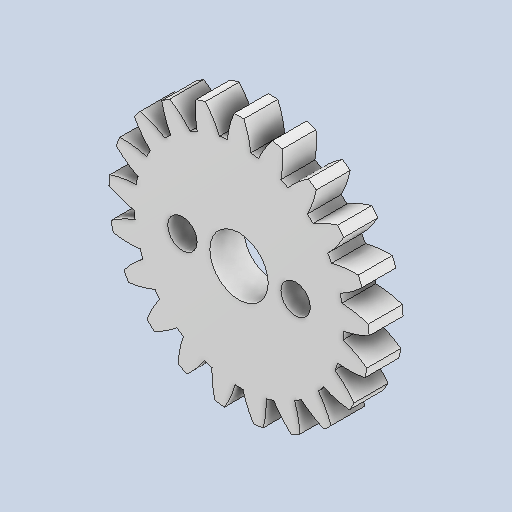
# Autodesk Inventor part: 平歯車1
Saved by Autodesk Inventor 2025.2 (Build 292293000, 293)
## iProperties
CustomPartVersion: 1
Created: 2025-01-07
Part Number: 平歯車1
Material: ABS プラスチック
Document SubType Name: Modeling
Designer: haruy
Categories: <?xml version="1.0" encoding="UTF-16"?> <MemberInstance><Categories><FamilyTemplate><FamilyTemplateParameter ValueType="xs:double" Id="1" ObjectReferenceKey="da_z" ObjectType="kUserParameterObject"/><FamilyTemplateParameter ValueType="xs:double" Id="2" ObjectReferenceKey="da_b" ObjectType="kUserParameterObject"/><FamilyTemplateParameter ValueType="xs:double" Id="3" ObjectReferenceKey="da_beta" ObjectType="kUserParameterObject"/><FamilyTemplateParameter ValueType="xs:double" Id="4" ObjectReferenceKey="da_da" ObjectType="kUserParameterObject"/><FamilyTemplateParameter ValueType="xs:double" Id="5" ObjectReferenceKey="da_aw" ObjectType="kUserParameterObject"/><FamilyTemplateParameter ValueType="xs:string" Id="6" ObjectReferenceKey="EAIAABAAAACIAQAAAAAAAIAAAAAAAAAA" ObjectType="83910656" SubObjectId="SurfaceGeometry"/></FamilyTemplate><ParamToTemplateMap><ParamToTemplate CategoryParameter="//CategoryParameter[@InternalName='046C89C9-8512-4d59-83FE-43B91F4F132A']" TemplateParameter="1"/><ParamToTemplate CategoryParameter="//CategoryParameter[@InternalName='2552DF32-E462-4b46-AEBF-C6C7768E72AC']" TemplateParameter="2"/><ParamToTemplate CategoryParameter="//CategoryParameter[@InternalName='C9EE641D-15FC-4fae-A226-E94C4372FDD7']" TemplateParameter="3"/><ParamToTemplate><ParamToTemplate CategoryParameter="//CategoryParameter[@InternalName='00B6519A-459B-49c7-AD84-2E56D39A5744']" ConstantValue="0.000000"/></ParamToTemplate><ParamToTemplate><ParamToTemplate CategoryParameter="//CategoryParameter[@InternalName='04B31F0E-C7A6-4894-AA32-9629BEFACF47']" ConstantValue="1.000000"/></ParamToTemplate><ParamToTemplate><ParamToTemplate CategoryParameter="//CategoryParameter[@InternalName='43CBEC2E-7847-49e7-A936-2F7889FCB2D9']" ConstantValue="0.250000"/></ParamToTemplate><ParamToTemplate><ParamToTemplate CategoryParameter="//CategoryParameter[@InternalName='B1EFC894-105D-4ebd-86BF-FA20ED196853']" ConstantValue="0.350000"/></ParamToTemplate><ParamToTemplate><ParamToTemplate CategoryParameter="//CategoryParameter[@InternalName='51175063-3D10-4879-93E8-6246FE8B403D']" ConstantValue="2060000000.000000"/></ParamToTemplate><ParamToTemplate><ParamToTemplate CategoryParameter="//CategoryParameter[@InternalName='A3A52E27-4454-46a9-B0BD-C932399B70AF']" ConstantValue="0.300000"/></ParamToTemplate><ParamToTemplate><ParamToTemplate CategoryParameter="//CategoryParameter[@InternalName='91B76062-C214-41d9-B1B9-14D2AB99603D']" ConstantValue="0.200000"/></ParamToTemplate><ParamToTemplate><ParamToTemplate CategoryParameter="//CategoryParameter[@InternalName='374E806E-8B8A-4dda-A9AA-1039D6500AD2']" ConstantValue="5.000000"/></ParamToTemplate><ParamToTemplate><ParamToTemplate CategoryParameter="//CategoryParameter[@InternalName='2D373A89-B862-43d6-8D0B-0CBF12AB9F6C']" ConstantValue="0.349066"/></ParamToTemplate><ParamToTemplate CategoryParameter="//CategoryParameter[@InternalName='37777632-D6A2-4fac-9D53-DB8ACD95C989']" TemplateParameter="4"/><ParamToTemplate CategoryParameter="//CategoryParameter[@InternalName='FD1017F1-B727-4f7e-9707-0F86F1FF9423']" TemplateParameter="5"/><ParamToTemplate><ParamToTemplate CategoryParameter="//CategoryParameter[@InternalName='9E1B4470-B2D3-4ff1-B813-535BB4CDF51A']" ConstantValue="3520000.000000"/></ParamToTemplate><ParamToTemplate><ParamToTemplate CategoryParameter="//CategoryParameter[@InternalName='F8452263-BFF6-458c-9FB1-07C4B99E95CD']" ConstantValue="11400000.000000"/></ParamToTemplate><ParamToTemplate><ParamToTemplate CategoryParameter="//CategoryParameter[@InternalName='3E3BB259-FD49-497f-8171-6EBC954A3479']" ConstantValue="2.000000"/></ParamToTemplate><ParamToTemplate CategoryParameter="//CategoryParameter[@InternalName='27C3BAF2-7550-4e4b-AE2C-0DB134B7D9B7']" TemplateParameter="6"/></ParamToTemplateMap><Category DisplayName="Gear" InternalName="DC85795E-93AB-48d5-8EEE-5A27447B64BD" Mnemonic="Gear"><CategoryParameter DisplayName="z" InternalName="046C89C9-8512-4d59-83FE-43B91F4F132A" Mnemonic="z"/><CategoryParameter DisplayName="b" InternalName="2552DF32-E462-4b46-AEBF-C6C7768E72AC" Mnemonic="b"/><CategoryParameter DisplayName="||b|" InternalName="C9EE641D-15FC-4fae-A226-E94C4372FDD7" Mnemonic="beta"/><CategoryParameter DisplayName="x" InternalName="00B6519A-459B-49c7-AD84-2E56D39A5744" Mnemonic="x"/><CategoryParameter DisplayName="a*" InternalName="04B31F0E-C7A6-4894-AA32-9629BEFACF47" Mnemonic="a"/><CategoryParameter DisplayName="c*" InternalName="43CBEC2E-7847-49e7-A936-2F7889FCB2D9" Mnemonic="c"/><CategoryParameter DisplayName="r|.f|*" InternalName="B1EFC894-105D-4ebd-86BF-FA20ED196853" Mnemonic="rf"/><CategoryParameter DisplayName="E" InternalName="51175063-3D10-4879-93E8-6246FE8B403D" Mnemonic="E"/><CategoryParameter DisplayName="||m|" InternalName="A3A52E27-4454-46a9-B0BD-C932399B70AF" Mnemonic="mi"/><Category DisplayName="SpurGear" InternalName="26C5A22E-A91E-4dfd-A3B3-23CCAFAE1764" Mnemonic="SpurGear"><CategoryParameter DisplayName="m" InternalName="91B76062-C214-41d9-B1B9-14D2AB99603D" Mnemonic="m"/><CategoryParameter DisplayName="P" InternalName="374E806E-8B8A-4dda-A9AA-1039D6500AD2" Mnemonic="PP"/><CategoryParameter DisplayName="||a|" InternalName="2D373A89-B862-43d6-8D0B-0CBF12AB9F6C" Mnemonic="alpha"/><CategoryParameter DisplayName="d|.a|" InternalName="37777632-D6A2-4fac-9D53-DB8ACD95C989" Mnemonic="da"/><CategoryParameter DisplayName="a|.w|" InternalName="FD1017F1-B727-4f7e-9707-0F86F1FF9423" Mnemonic="aw"/><CategoryParameter DisplayName="||s||.Flim|" InternalName="9E1B4470-B2D3-4ff1-B813-535BB4CDF51A" Mnemonic="sFlim"/><CategoryParameter DisplayName="||s||.Hlim|" InternalName="F8452263-BFF6-458c-9FB1-07C4B99E95CD" Mnemonic="sHlim"/><CategoryParameter DisplayName="タイプ" InternalName="3E3BB259-FD49-497f-8171-6EBC954A3479" Mnemonic="type"/><CategoryParameter DisplayName="PitchDiameter" InternalName="27C3BAF2-7550-4e4b-AE2C-0DB134B7D9B7" Mnemonic="IDS_PITCHDIAM"/></Category></Category></Categories></MemberInstance>
Density: 1.06 g/cm^3
Appearance: 滑らか - 白
Mass: 64.8659 g
Surface Area: 43.5022 cm^2
Volume: 8.26317 cm^3
Author: haruy
Autodesk Inventor part; units mm, degrees
sketch "Sketch1" plane through (0, 0, 0) normal (0, 0, 1) x (1, 0, 0)
  circle A0 centre (0, 0) radius 23
  dimension "d0" = 46
  constraints: 1 centre point
  measures "d0" diameter of A0
extrude "Extrusion1" add sketch "Sketch1" along normal blind 6
ref_plane "Work Plane2" through (0, 0, 3) normal (0, 0, 1) x (1, 0, 0)
sketch "Sketch2" plane through (0, 0, 0) normal (0, 0, -1) x (-1, 0, 0)
  circle A0 centre (0, 0) radius 23 projected
  circle A1 centre (0, 0) radius 21
  dimension "d3" = 42
  constraints: 1 centre point, 1 coincident
  measures "d3" diameter of A1
surface extrude "ピッチ円直径" sketch "Sketch2" against normal through all shown no curves A1
ref_plane "Work Plane8" through (0, 0, 0) normal (0.9888308, 0.1490423, 0) x (0, 0, 1)
ref_plane "Work Plane9" through (0, 0, 0) normal (1, 0, 0) x (0, 1, 0)
spur gear teeth "平歯車" teeth 21 pitch diameter 42 tip diameter 46 root diameter 37 face width 6 start plane through (0, 0, 0) normal (0, 0, -1) x (-1, 0, 0)
sketch "スケッチ3" plane through (0, 0, 6) normal (0, 0, 1) x (1, 0, 0)
  circle A0 centre (0, 0) radius 5.15
  circle A1 centre (0, 0) radius 10
  circle A2 centre (-10, 0) radius 2.6
  circle A3 centre (10, 0) radius 2.6
  dimension "d50" = 20
  dimension "d49" = 10.3
  dimension "d51" = 5.2
  dimension "d54" = 360
  constraints: 3 centre point, 2 coincident, 1 horizontal alignment, 7 other
  measures "d49" diameter of A0
  measures "d51" diameter of A2
extrude "押し出し2" cut sketch "スケッチ3" against normal blind 10 contours A0 | A1 A3 | A1 A3 | A2 A1 | A1 A2
sketch "スケッチ4" plane through (0, 0, 6) normal (0, 0, 1) x (1, 0, 0)
  circle A0 centre (10, 0) radius 2.6 projected
  circle A1 centre (-10, 0) radius 2.6 projected
  circle A2 centre (0, 0) radius 5.15 projected
  arc A3 (-5.9528, 22.2163) -> (-7.5964, 21.7093) centre (0, 0) ccw projected
  arc A4 (-7.5964, 21.7093) -> (-7.398, 16.9564) centre (9.3156, 20.0347) ccw projected
  arc A5 (-7.398, 16.9564) -> (-8.6445, 16.3561) centre (0, 0) ccw projected
  arc A6 (-8.6445, 16.3561) -> (-12.2367, 19.4747) centre (-21.472, 5.2082) ccw projected
  arc A7 (-12.2367, 19.4747) -> (-13.6579, 18.5057) centre (0, 0) ccw projected
  arc A8 (-13.6579, 18.5057) -> (-12.0673, 14.0225) centre (2.9964, 21.8905) ccw projected
  arc A9 (-12.0673, 14.0225) -> (-13.0815, 13.0815) centre (0, 0) ccw projected
  arc A10 (-13.0815, 13.0815) -> (-17.4333, 15.0026) centre (-22.0532, -1.3521) ccw projected
  arc A11 (-17.4333, 15.0026) -> (-18.5057, 13.6579) centre (0, 0) ccw projected
  arc A12 (-18.5057, 13.6579) -> (-15.6644, 9.8426) centre (-3.5891, 21.8011) ccw projected
  arc A13 (-15.6644, 9.8426) -> (-16.3561, 8.6445) centre (0, 0) ccw projected
  arc A14 (-16.3561, 8.6445) -> (-21.0809, 9.1975) centre (-20.6749, -7.7924) ccw projected
  arc A15 (-21.0809, 9.1975) -> (-21.7093, 7.5964) centre (0, 0) ccw projected
  arc A16 (-21.7093, 7.5964) -> (-17.8696, 4.7882) centre (-9.8556, 19.7747) ccw projected
  arc A17 (-17.8696, 4.7882) -> (-18.1775, 3.4394) centre (0, 0) ccw projected
  arc A18 (-18.1775, 3.4394) -> (-22.8554, 2.5752) centre (-17.4595, -13.5402) ccw projected
  arc A19 (-22.8554, 2.5752) -> (-22.9839, 0.86) centre (0, 0) ccw projected
  arc A20 (-22.9839, 0.86) -> (-18.4871, -0.6917) centre (-15.2464, 15.9912) ccw projected
  arc A21 (-18.4871, -0.6917) -> (-18.3837, -2.0713) centre (0, 0) ccw projected
  arc A22 (-18.3837, -2.0713) -> (-22.599, -4.276) centre (-12.6928, -18.0849) ccw projected
  arc A23 (-22.599, -4.276) -> (-22.2163, -5.9528) centre (0, 0) ccw projected
  arc A24 (-22.2163, -5.9528) -> (-17.4618, -6.1102) centre (-19.2826, 10.7868) ccw projected
  arc A25 (-17.4618, -6.1102) -> (-16.9564, -7.398) centre (0, 0) ccw projected
  arc A26 (-16.9564, -7.398) -> (-20.3347, -10.7472) centre (-6.7983, -21.0227) ccw projected
  arc A27 (-20.3347, -10.7472) -> (-19.4747, -12.2367) centre (0, 0) ccw projected
  arc A28 (-19.4747, -12.2367) -> (-14.8851, -10.9857) centre (-21.6053, 4.6239) ccw projected
  arc A29 (-14.8851, -10.9857) -> (-14.0225, -12.0673) centre (0, 0) ccw projected
  arc A30 (-14.0225, -12.0673) -> (-16.2635, -16.2635) centre (-0.2997, -22.0926) ccw projected
  arc A31 (-16.2635, -16.2635) -> (-15.0026, -17.4333) centre (0, 0) ccw projected
  arc A32 (-15.0026, -17.4333) -> (-10.9857, -14.8851) centre (-22.0084, -1.9498) ccw projected
  arc A33 (-10.9857, -14.8851) -> (-9.8426, -15.6644) centre (0, 0) ccw projected
  arc A34 (-9.8426, -15.6644) -> (-10.7472, -20.3347) centre (6.2255, -21.1994) ccw projected
  arc A35 (-10.7472, -20.3347) -> (-9.1975, -21.0809) centre (0, 0) ccw projected
  arc A36 (-9.1975, -21.0809) -> (-6.1102, -17.4618) centre (-20.4559, -8.3503) ccw projected
  arc A37 (-6.1102, -17.4618) -> (-4.7882, -17.8696) centre (0, 0) ccw projected
  arc A38 (-4.7882, -17.8696) -> (-4.276, -22.599) centre (12.1976, -18.4225) ccw projected
  arc A39 (-4.276, -22.599) -> (-2.5752, -22.8554) centre (0, 0) ccw projected
  arc A40 (-2.5752, -22.8554) -> (-0.6917, -18.4871) centre (-17.0858, -14.0088) ccw projected
  arc A41 (-0.6917, -18.4871) -> (0.6917, -18.4871) centre (0, 0) ccw projected
  arc A42 (0.6917, -18.4871) -> (2.5752, -22.8554) centre (17.0858, -14.0088) ccw projected
  arc A43 (2.5752, -22.8554) -> (4.276, -22.599) centre (0, 0) ccw projected
  arc A44 (4.276, -22.599) -> (4.7882, -17.8696) centre (-12.1976, -18.4225) ccw projected
  arc A45 (4.7882, -17.8696) -> (6.1102, -17.4618) centre (0, 0) ccw projected
  arc A46 (6.1102, -17.4618) -> (9.1975, -21.0809) centre (20.4559, -8.3503) ccw projected
  arc A47 (9.1975, -21.0809) -> (10.7472, -20.3347) centre (0, 0) ccw projected
  arc A48 (10.7472, -20.3347) -> (9.8426, -15.6644) centre (-6.2255, -21.1994) ccw projected
  arc A49 (9.8426, -15.6644) -> (10.9857, -14.8851) centre (0, 0) ccw projected
  arc A50 (10.9857, -14.8851) -> (15.0026, -17.4333) centre (22.0084, -1.9498) ccw projected
  arc A51 (15.0026, -17.4333) -> (16.2635, -16.2635) centre (0, 0) ccw projected
  arc A52 (16.2635, -16.2635) -> (14.0225, -12.0673) centre (0.2997, -22.0926) ccw projected
  arc A53 (14.0225, -12.0673) -> (14.8851, -10.9857) centre (0, 0) ccw projected
  arc A54 (14.8851, -10.9857) -> (19.4747, -12.2367) centre (21.6053, 4.6239) ccw projected
  arc A55 (19.4747, -12.2367) -> (20.3347, -10.7472) centre (0, 0) ccw projected
  arc A56 (20.3347, -10.7472) -> (16.9564, -7.398) centre (6.7983, -21.0227) ccw projected
  arc A57 (16.9564, -7.398) -> (17.4618, -6.1102) centre (0, 0) ccw projected
  arc A58 (17.4618, -6.1102) -> (22.2163, -5.9528) centre (19.2826, 10.7868) ccw projected
  arc A59 (22.2163, -5.9528) -> (22.599, -4.276) centre (0, 0) ccw projected
  arc A60 (22.599, -4.276) -> (18.3837, -2.0713) centre (12.6928, -18.0849) ccw projected
  arc A61 (18.3837, -2.0713) -> (18.4871, -0.6917) centre (0, 0) ccw projected
  arc A62 (18.4871, -0.6917) -> (22.9839, 0.86) centre (15.2464, 15.9912) ccw projected
  arc A63 (22.9839, 0.86) -> (22.8554, 2.5752) centre (0, 0) ccw projected
  arc A64 (22.8554, 2.5752) -> (18.1775, 3.4394) centre (17.4595, -13.5402) ccw projected
  arc A65 (18.1775, 3.4394) -> (17.8696, 4.7882) centre (0, 0) ccw projected
  arc A66 (17.8696, 4.7882) -> (21.7093, 7.5964) centre (9.8556, 19.7747) ccw projected
  arc A67 (21.7093, 7.5964) -> (21.0809, 9.1975) centre (0, 0) ccw projected
  arc A68 (21.0809, 9.1975) -> (16.3561, 8.6445) centre (20.6749, -7.7924) ccw projected
  arc A69 (16.3561, 8.6445) -> (15.6644, 9.8426) centre (0, 0) ccw projected
  arc A70 (15.6644, 9.8426) -> (18.5057, 13.6579) centre (3.5891, 21.8011) ccw projected
  arc A71 (18.5057, 13.6579) -> (17.4333, 15.0026) centre (0, 0) ccw projected
  arc A72 (17.4333, 15.0026) -> (13.0815, 13.0815) centre (22.0532, -1.3521) ccw projected
  arc A73 (13.0815, 13.0815) -> (12.0673, 14.0225) centre (0, 0) ccw projected
  arc A74 (12.0673, 14.0225) -> (13.6579, 18.5057) centre (-2.9964, 21.8905) ccw projected
  arc A75 (13.6579, 18.5057) -> (12.2367, 19.4747) centre (0, 0) ccw projected
  arc A76 (12.2367, 19.4747) -> (8.6445, 16.3561) centre (21.472, 5.2082) ccw projected
  arc A77 (8.6445, 16.3561) -> (7.398, 16.9564) centre (0, 0) ccw projected
  arc A78 (7.398, 16.9564) -> (7.5964, 21.7093) centre (-9.3156, 20.0347) ccw projected
  arc A79 (7.5964, 21.7093) -> (5.9528, 22.2163) centre (0, 0) ccw projected
  arc A80 (5.9528, 22.2163) -> (3.4394, 18.1775) centre (18.9829, 11.3058) ccw projected
  arc A81 (3.4394, 18.1775) -> (2.0713, 18.3837) centre (0, 0) ccw projected
  arc A82 (2.0713, 18.3837) -> (0.86, 22.9839) centre (-14.8071, 16.3988) ccw projected
  arc A83 (0.86, 22.9839) -> (-0.86, 22.9839) centre (0, 0) ccw projected
  arc A84 (-0.86, 22.9839) -> (-2.0713, 18.3837) centre (14.8071, 16.3988) ccw projected
  arc A85 (-2.0713, 18.3837) -> (-3.4394, 18.1775) centre (0, 0) ccw projected
  arc A86 (-3.4394, 18.1775) -> (-5.9528, 22.2163) centre (-18.9829, 11.3058) ccw projected
equation "\"d0\" = da_da"
equation "\"d1\" = da_b"
equation "\"d3\" = da_d"
equation "\"d16\" = da_aw"
equation "\"d43\" = da_aw"
equation "\"d46\" = da_aw"
equation "\"da_da\" = 46"
equation "\"da_b\" = 6"
equation "\"da_d\" = 42"
equation "\"da_aw\" = 42"
body "Solid1"
body "Srf1"
